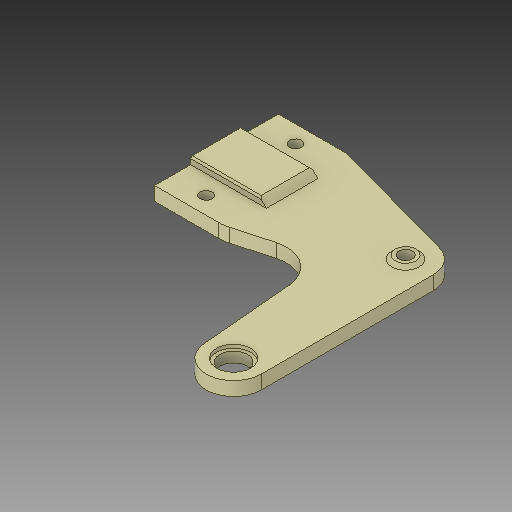
# Autodesk Inventor part: 04-06-Рычаг нижний
Saved by Autodesk Inventor 2018 (Build 220112000, 112)
## iProperties
Part Number: 04-06-Рычаг нижний
Material: Типовые
Document SubType Name: Modeling
Designer: sbnnl
Density: 1 g/cm^3
Appearance: Гладкий — пепельный
Author: sbnnl
Autodesk Inventor part; units mm, degrees
ref_plane "YZ Plane" through (0, 0, 0) normal (1, 0, 0) x (0, 1, 0)
ref_plane "XZ Plane" through (0, 0, 0) normal (0, 1, 0) x (-1, 0, 0)
ref_plane "XY Plane" through (0, 0, 0) normal (0, 0, 1) x (1, 0, 0)
sketch "Эскиз1" plane through (0, 0, 0) normal (0, 1, 0) x (-1, 0, 0)
  line L0 (0, 18) -> (0, -18)
  arc A0 (-57.1363, 7.7095) -> (-57.1363, -7.7095) centre (-55, 0) ccw
  line L1 (0, 0) -> (-6.25, 0) construction
  line L2 (0, 18) -> (-18.6401, 18)
  line L3 (-21.3105, 17.6369) -> (-57.1363, 7.7095)
  line L4 (0, -18) -> (-18.6401, -18)
  line L5 (-21.3105, -17.6369) -> (-57.1363, -7.7095)
  circle A1 centre (-55, 0) radius 2
  arc A2 (-18.6401, 18) -> (-21.3105, 17.6369) centre (-18.6401, 8) ccw
  arc A3 (-21.3105, -17.6369) -> (-18.6401, -18) centre (-18.6401, -8) ccw
  circle A4 centre (-10, -13) radius 1.75
  circle A5 centre (-10, 13) radius 1.75
  line L6 (-10, 13) -> (-10, -13) construction
  point P0 (-20, 18)
  dimension "d0" = 16
  dimension "d1" = 36
  dimension "d2" = 55
  dimension "d3" = 20
  dimension "d4" = 4
  dimension "d5" = 10
  dimension "d18" = 3.5
  dimension "d19" = 13
  dimension "d20" = 10
  constraints: 14 end point, 6 centre point, 6 point on circle, 6 tangent, 3 horizontal, 3 point on line, 2 vertical, 1 coincident, 1 equal radius, 1 midpoint, 1 parallel, 1 symmetric about line, 1 other
  measures "d0" diameter of A0
  measures "d1" distance of L0.start L0.end
  measures "d2" distance from line of L0 A0.centre
  measures "d3" distance of L0.start point (-20, 18)
  measures "d4" diameter of A1
  measures "d5" radius of A2
  measures "d18" diameter of A4
  measures "d19" distance from line of L6.end L1
  measures "d20" distance between parallel lines of L6 L0
extrude "Выдавливание1" add sketch "Эскиз1" along normal blind 4
sketch "Эскиз2" plane through (0, 4, 0) normal (0, 1, 0) x (1, 0, 0)
  line L0 (0, 0) -> (14.985, 0) construction
  line L1 (0, 7.5) -> (22, 7.5)
  line L2 (22, 7.5) -> (22, -7.5)
  line L3 (22, -7.5) -> (0, -7.5)
  line L4 (0, -7.5) -> (0, 7.5)
  line L5 (0, 18) -> (0, -18) projected
  dimension "d8" = 15
  dimension "d9" = 22
  constraints: 10 end point, 2 horizontal, 2 parallel, 1 collinear, 1 perpendicular, 1 other
  measures "d8" distance of L3.end L1.start
  measures "d9" distance of L1.start L1.end
extrude "Выдавливание2" add sketch "Эскиз2" along normal blind 2
chamfer "Фаска1" distance 2 angle 45 1 edges at (22, 6, 0)
chamfer "Фаска2" distance 0.5 angle 45 2 edges at (10.0002, 6, 7.5) (10.0003, 6, -7.5)
sketch "Эскиз4" plane through (0, 4, 0) normal (0, 1, 0) x (1, 0, 0)
  arc A0 (47.0304, -50.6972) -> (63, -50) centre (55, -50) ccw
  line L0 (63, -50) -> (63, 0)
  arc A1 (57.1363, -7.7095) -> (57.1363, 7.7095) centre (55, 0) ccw projected
  line L1 (47.0304, -50.6972) -> (43.5977, -11.461)
  line L2 (57.1363, -7.7095) -> (21.3105, -17.6369) projected
  circle A2 centre (55, -50) radius 4
  point P0 (0, 0)
  dimension "d21" = 16
  dimension "d22" = 50
  dimension "d23" = 55
  dimension "d24" = 5
  dimension "d34" = 8
  dimension "d35" = 55
  constraints: 4 end point, 3 point on circle, 3 tangent, 2 centre point, 1 coincident, 1 point on line
  measures "d21" diameter of A0
  measures "d22" vertical distance of A0.centre point (0, 0)
  measures "d23" horizontal distance of A0.centre point (0, 0)
  measures "d24" angle of L1 L0
  measures "d34" diameter of A2
  measures "d35" distance of A1.centre point (0, 0)
extrude "Выдавливание3" add sketch "Эскиз4" against normal up to surface (4 mm away)
fillet "Сопряжение1" radius 10 1 edges at (43.5977, 2, 11.461)
sketch "Эскиз5" plane through (0, 4, 0) normal (0, 1, 0) x (1, 0, 0)
  circle A0 centre (55, 0) radius 2 projected
  circle A1 centre (55, 0) radius 3
  point P0 (0, 0)
  dimension "d28" = 1
  constraints: 1 centre point
  measures "d28" radial gap between concentric circles of A0 A1
extrude "Выдавливание4" add sketch "Эскиз5" along normal blind 1
chamfer "Фаска3" distance 1 angle 45 1 edges at (52, 4, 0)
sketch "Эскиз7" plane through (0, 4, 0) normal (0, 1, 0) x (1, 0, 0)
  circle A0 centre (55, -50) radius 4 projected
  circle A1 centre (55, -50) radius 5
  point P0 (0, 0)
  dimension "d36" = 10
  constraints: 1 centre point, 1 coincident
  measures "d36" diameter of A1
extrude "Выдавливание5" cut sketch "Эскиз7" against normal blind 1
